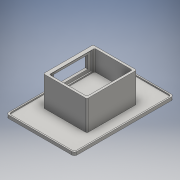
# Autodesk Inventor part: sampleChamberExt_v1
Saved by Autodesk Inventor 2016 (Build 200138000, 138)
## iProperties
Created: 2016-11-04
Part Number: sampleChamberExt_v1
Material: Generic
Document SubType Name: Modeling
Designer: sims01
Density: 1 g/cm^3
Appearance: Default
Author: sims01
Autodesk Inventor part; units mm, degrees
ref_plane "YZ Plane" through (0, 0, 0) normal (1, 0, 0) x (0, 1, 0)
ref_plane "XZ Plane" through (0, 0, 0) normal (0, 1, 0) x (-1, 0, 0)
ref_plane "XY Plane" through (0, 0, 0) normal (0, 0, 1) x (1, 0, 0)
sketch "Sketch1" plane through (0, 0, 0) normal (0, 0, 1) x (1, 0, 0)
  line L0 (-50.75, 79.75) -> (50.75, 79.75)
  line L1 (54.75, 75.75) -> (54.75, -75.75)
  line L2 (50.75, -79.75) -> (-50.75, -79.75)
  line L3 (-54.75, -75.75) -> (-54.75, 75.75)
  arc A0 (-50.75, 79.75) -> (-54.75, 75.75) centre (-50.75, 75.75) ccw
  arc A1 (-54.75, -75.75) -> (-50.75, -79.75) centre (-50.75, -75.75) ccw
  arc A2 (50.75, -79.75) -> (54.75, -75.75) centre (50.75, -75.75) ccw
  arc A3 (54.75, 75.75) -> (50.75, 79.75) centre (50.75, 75.75) ccw
  point P0 (0, 0)
  point P1 (-54.75, 79.75)
  point P2 (54.75, 79.75)
  point P3 (-54.75, -79.75)
  dimension "d0" = 109.5
  dimension "d1" = 159.5
  dimension "d2" = 54.75
  dimension "d3" = 79.75
  dimension "d4" = 4
  constraints: 8 end point, 8 point on circle, 8 tangent, 6 point on line, 4 centre point, 3 equal radius, 2 parallel, 1 horizontal, 1 perpendicular
  measures "d0" distance of point (-54.75, 79.75) point (54.75, 79.75)
  measures "d1" distance of point (-54.75, -79.75) point (-54.75, 79.75)
  measures "d2" distance from line of point (0, 0) L1
  measures "d3" distance from line of point (0, 0) L0
  measures "d4" radius of A0
extrude "xyAttach" add sketch "Sketch1" along normal blind 3
sketch "Sketch2" plane through (0, 0, 3) normal (0, 0, 1) x (1, 0, 0)
  line L0 (-50.75, 79.75) -> (50.75, 79.75)
  line L1 (54.75, 75.75) -> (54.75, -75.75)
  line L2 (50.75, -79.75) -> (-50.75, -79.75)
  line L3 (-54.75, -75.75) -> (-54.75, 75.75)
  line L4 (50.75, 79.75) -> (-50.75, 79.75) projected
  line L5 (-54.75, 75.75) -> (-54.75, -75.75) projected
  line L6 (-50.75, -79.75) -> (50.75, -79.75) projected
  line L7 (54.75, -75.75) -> (54.75, 75.75) projected
  arc A0 (-50.75, 79.75) -> (-54.75, 75.75) centre (-50.75, 75.75) ccw
  arc A1 (-54.75, -75.75) -> (-50.75, -79.75) centre (-50.75, -75.75) ccw
  arc A2 (50.75, -79.75) -> (54.75, -75.75) centre (50.75, -75.75) ccw
  arc A3 (54.75, 75.75) -> (50.75, 79.75) centre (50.75, 75.75) ccw
  line L8 (-48.75, 77.75) -> (48.75, 77.75)
  line L9 (52.75, 73.75) -> (52.75, -73.75)
  line L10 (48.75, -77.75) -> (-48.75, -77.75)
  line L11 (-52.75, -73.75) -> (-52.75, 73.75)
  arc A4 (-48.75, 77.75) -> (-52.75, 73.75) centre (-48.75, 73.75) ccw
  arc A5 (-52.75, -73.75) -> (-48.75, -77.75) centre (-48.75, -73.75) ccw
  arc A6 (48.75, -77.75) -> (52.75, -73.75) centre (48.75, -73.75) ccw
  arc A7 (52.75, 73.75) -> (48.75, 77.75) centre (48.75, 73.75) ccw
  point P0 (0, 0)
  dimension "d7" = 4
  dimension "d8" = 4
  dimension "d9" = 2
  dimension "d10" = 2
  dimension "d11" = 2
  dimension "d12" = 2
  constraints: 16 end point, 16 point on circle, 16 tangent, 8 centre point, 6 equal radius, 4 collinear, 4 parallel, 2 horizontal, 2 perpendicular
  measures "d7" radius of A0
  measures "d8" radius of A4
  measures "d9" distance between parallel lines of L8 L0
  measures "d10" distance between parallel lines of L3 L11
  measures "d11" distance between parallel lines of L2 L10
  measures "d12" distance between parallel lines of L1 L9
extrude "spillExtrusion" add sketch "Sketch2" along normal blind 2
sketch "Sketch3" plane through (0, 0, 3) normal (0, 0, 1) x (1, 0, 0)
  line L0 (-33, 40) -> (33, 40)
  line L1 (35, 38) -> (35, -38)
  line L2 (33, -40) -> (-33, -40)
  line L3 (-35, -38) -> (-35, 38)
  arc A0 (-33, 40) -> (-35, 38) centre (-33, 38) ccw
  arc A1 (-35, -38) -> (-33, -40) centre (-33, -38) ccw
  arc A2 (35, 38) -> (33, 40) centre (33, 38) ccw
  arc A3 (33, -40) -> (35, -38) centre (33, -38) ccw
  point P0 (0, 0)
  point P1 (-35, 40)
  point P2 (35, -40)
  point P3 (35, 40)
  dimension "d15" = 70
  dimension "d16" = 35
  dimension "d17" = 80
  dimension "d18" = 40
  dimension "d19" = 2
  constraints: 8 end point, 8 point on circle, 8 tangent, 6 point on line, 4 centre point, 3 equal radius, 2 parallel, 1 horizontal, 1 perpendicular
  measures "d15" distance of point (-35, 40) point (35, 40)
  measures "d16" distance from line of point (0, 0) L1
  measures "d17" distance of point (35, 40) point (35, -40)
  measures "d18" distance from line of point (0, 0) L0
  measures "d19" radius of A0
extrude "chamberWallExtrusion" add sketch "Sketch3" along normal blind 47.5
sketch "Sketch4" plane through (0, 0, 50.5) normal (0, 0, 1) x (1, 0, 0)
  line L0 (-27, 36.5) -> (29.5, 36.5)
  line L1 (31.5, 34.5) -> (31.5, -34.5)
  line L2 (29.5, -36.5) -> (-27, -36.5)
  line L3 (-29, -34.5) -> (-29, 34.5)
  arc A0 (-27, 36.5) -> (-29, 34.5) centre (-27, 34.5) ccw
  arc A1 (-29, -34.5) -> (-27, -36.5) centre (-27, -34.5) ccw
  arc A2 (29.5, -36.5) -> (31.5, -34.5) centre (29.5, -34.5) ccw
  arc A3 (31.5, 34.5) -> (29.5, 36.5) centre (29.5, 34.5) ccw
  line L4 (33, 40) -> (-33, 40) projected
  line L5 (35, -38) -> (35, 38) projected
  line L6 (-33, -40) -> (33, -40) projected
  line L7 (-35, 38) -> (-35, -38) projected
  point P0 (0, 0)
  dimension "d22" = 2
  dimension "d23" = 3.5
  dimension "d24" = 3.5
  dimension "d25" = 3.5
  dimension "d26" = 6
  constraints: 8 end point, 8 point on circle, 8 tangent, 4 centre point, 3 equal radius, 2 parallel, 1 horizontal, 1 perpendicular
  measures "d22" radius of A0
  measures "d23" distance between parallel lines of L0 L4
  measures "d24" distance between parallel lines of L5 L1
  measures "d25" distance between parallel lines of L6 L2
  measures "d26" distance between parallel lines of L7 L3
extrude "chamberInteriorExtrusion" cut sketch "Sketch4" against normal blind 32.5
sketch "Sketch5" plane through (-29, -34.5, 50.5) normal (1, 0, 0) x (0, 0, -1)
  line L0 (0.5, 2) -> (30.5, 2)
  line L1 (30.5, 2) -> (30.5, 67)
  line L2 (30.5, 67) -> (0.5, 67)
  line L3 (0.5, 67) -> (0.5, 2)
  line L4 (45.5, 110.25) -> (45.5, -41.25) projected
  point P0 (50.5, 34.5)
  dimension "d29" = 65
  dimension "d30" = 30
  dimension "d31" = 32.5
  dimension "d32" = 45
  constraints: 8 end point, 2 parallel, 1 horizontal, 1 perpendicular
  measures "d29" distance of L2.end L0.start
  measures "d30" distance of L1.end L2.end
  measures "d31" distance from line of L2 point (50.5, 34.5)
  measures "d32" distance between parallel lines of L4 L3
extrude "rectCoverSlipMountExtrusion" cut sketch "Sketch5" against normal blind 2
sketch "Sketch6" plane through (-31, -34.5, 50.5) normal (1, 0, 0) x (0, 0, -1)
  line L0 (5.5, 7) -> (25.5, 7)
  line L1 (25.5, 7) -> (25.5, 62)
  line L2 (25.5, 62) -> (5.5, 62)
  line L3 (5.5, 62) -> (5.5, 7)
  line L4 (45.5, -39.25) -> (45.5, 108.25) projected
  point P0 (50.5, 34.5)
  dimension "d35" = 55
  dimension "d36" = 20
  dimension "d37" = 40
  dimension "d38" = 27.5
  constraints: 8 end point, 2 parallel, 1 horizontal, 1 perpendicular
  measures "d35" distance of L2.end L0.start
  measures "d36" distance of L1.end L2.end
  measures "d37" distance between parallel lines of L4 L3
  measures "d38" distance from line of L2 point (50.5, 34.5)
extrude "rectCoverSlipWindow" cut sketch "Sketch6" against normal up to surface (4 mm away)
equation "\"d2\" = 0.5 * d0"
equation "\"d3\" = 0.5 * d1"
equation "\"d10\" = d9"
equation "\"d11\" = d9"
equation "\"d12\" = d9"
equation "\"d16\" = 0.5 * d15"
equation "\"d18\" = 0.5 * d17"
equation "\"d24\" = d23"
equation "\"d25\" = d23"
equation "\"d31\" = 0.5 * d29"
equation "\"d38\" = 0.5 * d35"
body "Solid1"
